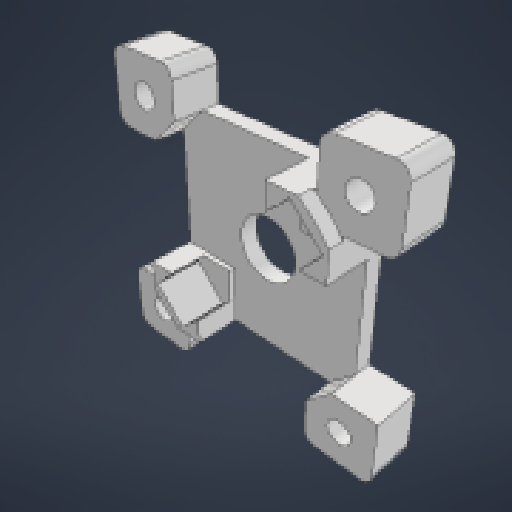
# Autodesk Inventor part: SistemaLiberacion2.2
Saved by Autodesk Inventor 2026.1 (Build 301233000, 233)
## iProperties
Created: 2025-11-13
Part Number: SistemaLiberacion2.2
Material: PLA
Document SubType Name: Modeling
Designer: usuario
Density: 1.3 g/cm^3
Appearance: Genérico
Mass: 76.0734 g
Surface Area: 228.636 cm^2
Volume: 58.518 cm^3
Author: usuario
Autodesk Inventor part; units mm, degrees
ref_plane "YZ Plane" through (0, 0, 0) normal (1, 0, 0) x (0, 1, 0)
ref_plane "XZ Plane" through (0, 0, 0) normal (0, 1, 0) x (-1, 0, 0)
ref_plane "XY Plane" through (0, 0, 0) normal (0, 0, 1) x (1, 0, 0)
sketch "Boceto1" plane through (0, 0, 0) normal (0, 0, 1) x (1, 0, 0)
  line L0 (-49, 49) -> (-49, -49)
  line L1 (-49, -49) -> (49, -49)
  line L2 (49, -49) -> (49, 49)
  line L3 (49, 49) -> (-49, 49)
  line L4 (-49, 49) -> (49, -49) construction
  line L5 (-49, -49) -> (49, 49) construction
  line L6 (-43, 43) -> (-43, -43)
  line L7 (-43, -43) -> (43, -43)
  line L8 (43, -43) -> (43, 43)
  line L9 (43, 43) -> (-43, 43)
  line L10 (-43, 43) -> (43, -43) construction
  line L11 (-43, -43) -> (43, 43) construction
  line L12 (-49, -30) -> (49, -30)
  line L13 (-49, 30) -> (49, 30)
  line L14 (-30, -49) -> (-30, 49)
  line L15 (30, -49) -> (30, 49)
  point P0 (0, 0)
  point P1 (0, -30)
  point P2 (0, -49)
  point P3 (-30, 43)
  point P4 (-43, 30)
  point P5 (30, 43)
  point P6 (43, 30)
  point P7 (30, -43)
  point P8 (43, -30)
  point P9 (-30, -43)
  point P10 (-43, -30)
  dimension "d0" = 98
  dimension "d1" = 98
  dimension "d2" = 6
  dimension "d3" = 6
  dimension "d8" = 19
  dimension "d10" = 19
  dimension "d11" = 19
  dimension "d18" = 19
  constraints: 32 end point, 8 point on line, 6 midpoint, 6 perpendicular, 4 parallel, 1 vertical
  measures "d0" distance of L0.start L0.end
  measures "d1" distance of L1.end L0.end
  measures "d2" distance between parallel lines of L1 L7
  measures "d3" distance between parallel lines of L8 L2
  measures "d8" distance of point (0, -30) point (0, -49)
  measures "d10" distance between parallel lines of L14 L0
  measures "d11" distance between parallel lines of L2 L15
  measures "d18" distance between parallel lines of L3 L13
extrude "Extrusión1" add sketch "Boceto1" against normal blind 34 contours L3 L14 L9 L6 L13 L0 | L12 L6 L7 L14 L1 L0 | L3 L2 L13 L8 L9 L15 | L15 L7 L8 L12 L2 L1
sketch "Boceto2" plane through (0, 0, -34) normal (0, 0, -1) x (-1, 0, 0)
  circle A0 centre (0, 0) radius 10.5
  line L0 (30, -49) -> (49, -49) projected
  line L1 (-49, 49) -> (-49, 30) projected
  line L2 (49, -49) -> (-49, -49)
  line L3 (-49, -49) -> (-49, 49)
  line L4 (-49, 49) -> (49, 49)
  line L5 (49, 49) -> (49, -49)
  line L6 (25, -49) -> (-25, -49)
  line L7 (-25, -49) -> (-25, -33.5)
  line L8 (-25, -33.5) -> (25, -33.5)
  line L9 (25, -33.5) -> (25, -49)
  line L10 (25, -49) -> (-25, -33.5) construction
  line L11 (-25, -49) -> (25, -33.5) construction
  line L12 (49, 0) -> (-49, 0) construction
  line L13 (0, -49) -> (0, 49) construction
  line L14 (33.5, -25) -> (33.5, 25)
  line L15 (49, 25) -> (33.5, -25) construction
  line L16 (49, -25) -> (33.5, -25)
  line L17 (49, 25) -> (49, -25)
  line L18 (49, -25) -> (33.5, 25) construction
  line L19 (33.5, 25) -> (49, 25)
  line L20 (25, 33.5) -> (-25, 33.5)
  line L21 (-25, 49) -> (25, 33.5) construction
  line L22 (25, 49) -> (25, 33.5)
  line L23 (-25, 49) -> (25, 49)
  line L24 (25, 49) -> (-25, 33.5) construction
  line L25 (-25, 33.5) -> (-25, 49)
  line L26 (-33.5, 25) -> (-33.5, -25)
  line L27 (-49, -25) -> (-33.5, 25) construction
  line L28 (-49, 25) -> (-33.5, 25)
  line L29 (-49, -25) -> (-49, 25)
  line L30 (-49, 25) -> (-33.5, -25) construction
  line L31 (-33.5, -25) -> (-49, -25)
  point P0 (0, -41.25)
  point P1 (-25, -49)
  point P2 (49, 0)
  point P3 (41.25, 0)
  point P4 (0, 49)
  point P5 (0, 41.25)
  point P6 (-49, 0)
  point P7 (-41.25, 0)
  dimension "d28" = 21
  dimension "d65" = 50
  dimension "d66" = 15.5
  dimension "d82" = 360
  constraints: 60 end point, 5 midpoint, 4 parallel, 2 horizontal, 2 perpendicular, 1 centre point, 1 coincident, 1 collinear, 1 point on line, 49 other
  measures "d28" diameter of A0
  measures "d65" distance of L7.end L8.end
  measures "d66" distance of L6.end L7.end
extrude "Extrusión2" add sketch "Boceto2" along normal blind 6 contours L2 L9 L8 L7 L3 L31 L26 L28 L1 L4 L25 L20 L22 L5 L19 L14 L16 L0
sketch "Boceto3" plane through (0, 0, -34) normal (0, 0, 1) x (1, 0, 0)
  line L0 (30, -49) -> (-30, -49) projected
  line L1 (-49, -30) -> (-49, 30) projected
  line L2 (-25, -49) -> (-49, -49)
  line L3 (-49, -49) -> (-49, -25)
  line L4 (-49, -25) -> (-33.5, -25)
  line L5 (-25, -33.5) -> (-25, -49)
  line L6 (30, 43) -> (30, 49) projected
  line L7 (25, 49) -> (30, 49) projected
  line L8 (-30, 49) -> (-30, 43) projected
  line L9 (-30, 43) -> (-43, 43) projected
  line L10 (-43, 43) -> (-43, 30) projected
  line L11 (-43, 30) -> (-49, 30) projected
  line L12 (-49, 25) -> (-49, 30) projected
  line L13 (-49, -30) -> (-43, -30) projected
  line L14 (-43, -30) -> (-43, -43) projected
  line L15 (-43, -43) -> (-30, -43) projected
  line L16 (-30, -43) -> (-30, -49) projected
  line L17 (-25, -49) -> (-30, -49) projected
  line L18 (30, -49) -> (30, -43) projected
  line L19 (30, -43) -> (43, -43) projected
  line L20 (43, -43) -> (43, -30) projected
  line L21 (43, -30) -> (49, -30) projected
  line L22 (49, -25) -> (49, -30) projected
  line L23 (49, 30) -> (43, 30) projected
  line L24 (43, 30) -> (43, 43) projected
  line L25 (43, 43) -> (30, 43) projected
  circle A0 centre (0, 0) radius 10.5 projected
  line L26 (-25, -33.5) -> (-13.5, -33.5)
  line L27 (-13.5, -33.5) -> (-13.5, -13.5)
  line L28 (-13.5, -13.5) -> (-33.5, -13.5)
  line L29 (-33.5, -13.5) -> (-33.5, -25)
  line L30 (-13.5, -29.5) -> (-29.5, -13.5)
  circle A1 centre (0, 0) radius 10.5 projected
  line L31 (13.5, 13.5) -> (33.5, 13.5)
  line L32 (13.5, 33.5) -> (13.5, 13.5)
  line L33 (13.5, 29.5) -> (29.5, 13.5)
  line L34 (33.5, 13.5) -> (33.5, 25)
  line L35 (25, 33.5) -> (13.5, 33.5)
  line L36 (25, 49) -> (49, 49)
  line L37 (49, 49) -> (49, 25)
  line L38 (49, 25) -> (33.5, 25)
  line L39 (25, 33.5) -> (25, 49)
  line L40 (25, 33.5) -> (25, 49) projected
  line L41 (-25, 33.5) -> (25, 33.5) projected
  line L42 (-25, 49) -> (-25, 33.5) projected
  line L43 (-30, 49) -> (-25, 49) projected
  line L44 (-33.5, 25) -> (-49, 25) projected
  line L45 (-33.5, -25) -> (-33.5, 25) projected
  line L46 (-49, -25) -> (-33.5, -25) projected
  line L47 (-49, -30) -> (-49, -25) projected
  line L48 (-25, -33.5) -> (-25, -49) projected
  line L49 (25, -33.5) -> (-25, -33.5) projected
  line L50 (25, -49) -> (25, -33.5) projected
  line L51 (30, -49) -> (25, -49) projected
  line L52 (33.5, -25) -> (49, -25) projected
  line L53 (33.5, 25) -> (33.5, -25) projected
  line L54 (49, 25) -> (33.5, 25) projected
  line L55 (49, 30) -> (49, 25) projected
  line L56 (-49, -30) -> (-49, -49) projected
  line L57 (33.5, -25) -> (25, -33.5)
  line L58 (-25, 33.5) -> (-33.5, 25)
  point P0 (49, 49)
  point P1 (30, 49)
  point P2 (49, 30)
  point P3 (49, 25)
  point P4 (49, 30)
  point P5 (43, 30)
  point P6 (43, 43)
  point P7 (30, 43)
  point P8 (30, 49)
  dimension "d74" = 4
  dimension "d77" = 360
  dimension "d84" = 45
  dimension "d85" = 20
  dimension "d86" = 20
  constraints: 40 end point, 4 collinear, 4 parallel, 4 point on line, 2 horizontal, 2 perpendicular, 53 other
  measures "d74" distance of L28.end L30.end
  measures "d84" angle of L30 L45
  measures "d85" distance of L26.end L27.end
  measures "d86" distance of L27.end L28.end
extrude "Extrusión3" add sketch "Boceto3" along normal blind 15 contours L0 L50 L57 L52 L22 L21 L20 L19 L18 | L0 L16 L15 L14 L13 L1 L4 L29 L28 L30 L27 L26 L5 | L30 L28 L27 | L31 L33 L32 L35 L39 L7 L6 L25 L24 L23 L37 L38 L34 | L31 L32 L33 | L1 L11 L10 L9 L8 L43 L42 L58 L44
sketch "Boceto4" plane through (0, 0, -19) normal (0, 0, 1) x (1, 0, 0)
  line L0 (30, 49) -> (30, 43) projected
  line L1 (43, 43) -> (43, 30) projected
  line L2 (30, 43) -> (43, 43) projected
  line L3 (-18.7383, -7.4246) -> (-27.9307, -16.617)
  line L4 (-27.9307, -16.617) -> (-16.617, -27.9307)
  line L5 (-16.617, -27.9307) -> (-7.4246, -18.7383)
  line L6 (-7.4246, -18.7383) -> (-18.7383, -7.4246)
  line L7 (-16.617, -27.9307) -> (-18.7383, -7.4246) construction
  line L8 (-27.9307, -16.617) -> (-7.4246, -18.7383) construction
  circle A0 centre (0, 0) radius 10.5 construction
  line L9 (18.7383, 7.4246) -> (27.9307, 16.617)
  line L10 (27.9307, 16.617) -> (16.617, 27.9307)
  line L11 (16.617, 27.9307) -> (18.7383, 7.4246) construction
  line L12 (27.9307, 16.617) -> (7.4246, 18.7383) construction
  line L13 (7.4246, 18.7383) -> (18.7383, 7.4246)
  line L14 (16.617, 27.9307) -> (7.4246, 18.7383)
  line L15 (49, -49) -> (25, -49) construction
  line L16 (-49, -49) -> (-49, 49) construction
  line L17 (49, -49) -> (-49, -49) construction
  line L18 (-49, -49) -> (-49, 49) construction
  line L19 (-49, 49) -> (49, 49) construction
  line L20 (49, 49) -> (49, -49) construction
  line L21 (49, -49) -> (-49, -49) construction
  line L22 (49, 49) -> (-49, -49) construction
  line L23 (-49, 49) -> (49, -49) construction
  point P0 (0, 0)
  point P1 (-17.6777, -17.6777)
  point P2 (17.6777, 17.6777)
  point P3 (-17.6777, -17.6777)
  point P4 (-49, 25)
  point P5 (-25, -49)
  dimension "d54" = 13
  dimension "d57" = 16
  dimension "d61" = 360
  dimension "d64" = 25
  dimension "d79" = 8
  constraints: 36 end point, 4 perpendicular, 2 midpoint, 2 parallel, 1 coincident, 1 horizontal, 1 point on line, 23 other
  measures "d54" distance of L3.start L3.end
  measures "d57" distance of L3.end L4.end
  measures "d64" distance of point (0, 0) point (-17.678, -17.678)
  measures "d79" distance between parallel lines of L22 L3
extrude "Extrusión4" cut sketch "Boceto4" against normal blind 13
sketch "Boceto6" plane through (0, 0, 0) normal (0, 0, 1) x (1, 0, 0)
  line L0 (-49, -49) -> (-30, -49) projected
  line L1 (-49, -30) -> (-49, -49) projected
  line L2 (-49, 49) -> (-49, 30) projected
  line L3 (-30, 49) -> (-49, 49) projected
  line L4 (49, 49) -> (30, 49) projected
  line L5 (49, 30) -> (49, 49) projected
  line L6 (30, -49) -> (49, -49) projected
  line L7 (49, -49) -> (49, -30) projected
  line L8 (-43, -43) -> (-43, -30) projected
  line L9 (-30, -43) -> (-43, -43) projected
  line L10 (-43, 30) -> (-43, 43) projected
  line L11 (-43, 43) -> (-30, 43) projected
  line L12 (30, 43) -> (43, 43) projected
  line L13 (43, 43) -> (43, 30) projected
  line L14 (43, -30) -> (43, -43) projected
  line L15 (43, -43) -> (30, -43) projected
  line L16 (-43, -43) -> (43, -43)
  line L17 (43, -43) -> (43, 43)
  line L18 (43, 43) -> (-43, 43)
  line L19 (-43, 43) -> (-43, -43)
  line L20 (-49, -49) -> (49, -49)
  line L21 (49, -49) -> (49, 49)
  line L22 (49, 49) -> (-49, 49)
  line L23 (-49, 49) -> (-49, -49)
  point P0 (0, 0)
  constraints: 16 end point, 4 parallel, 2 horizontal, 2 perpendicular
extrude "Extrusión5" cut sketch "Boceto6" against normal blind 11
sketch "Boceto8" plane through (0, 0, -19) normal (0, 0, 1) x (1, 0, 0)
  line L0 (-49, 49) -> (-25, 49) construction
  line L1 (49, -49) -> (25, -49) construction
  line L2 (-49, 49) -> (49, 49) construction
  line L3 (49, 49) -> (49, -49) construction
  line L4 (49, -49) -> (-49, -49) construction
  line L5 (-49, -49) -> (-49, 49) construction
  line L6 (-49, 49) -> (49, -49) construction
  line L7 (49, 49) -> (-49, -49) construction
  line L8 (-27.6832, -16.8645) -> (-31.9259, -21.1071)
  line L9 (-31.9259, -21.1071) -> (-21.1071, -31.9259)
  line L10 (-27.6832, -16.8645) -> (-16.8645, -27.6832)
  line L11 (-16.8645, -27.6832) -> (-21.1071, -31.9259)
  line L12 (-27.6832, -16.8645) -> (-21.1071, -31.9259) construction
  line L13 (-31.9259, -21.1071) -> (-16.8645, -27.6832) construction
  line L14 (-16.617, -27.9307) -> (-27.9307, -16.617) construction
  line L15 (-31.9259, -21.1071) -> (-23.4406, -12.6219) construction
  line L16 (-23.4406, -12.6219) -> (-12.6219, -23.4406) construction
  line L17 (-12.6219, -23.4406) -> (-21.1071, -31.9259) construction
  circle A0 centre (0, 0) radius 10.5 projected
  line L18 (27.6832, 16.8645) -> (16.8645, 27.6832)
  line L19 (31.9259, 21.1071) -> (16.8645, 27.6832) construction
  line L20 (31.9259, 21.1071) -> (21.1071, 31.9259)
  line L21 (27.6832, 16.8645) -> (21.1071, 31.9259) construction
  line L22 (16.8645, 27.6832) -> (21.1071, 31.9259)
  line L23 (27.6832, 16.8645) -> (31.9259, 21.1071)
  point P0 (-24.3952, -24.3952)
  point P1 (24.3952, 24.3952)
  point P2 (23.4406, 12.6219)
  dimension "d87" = 6
  dimension "d88" = 15.3
  dimension "d89" = 12
  dimension "d94" = 360
  constraints: 42 end point, 4 parallel, 4 perpendicular, 3 point on line, 2 collinear, 1 horizontal, 1 midpoint, 25 other
  measures "d87" distance of L8.start L8.end
  measures "d88" distance of L8.end L9.end
  measures "d89" distance of L8.end L15.end
extrude "Extrusión7" cut sketch "Boceto8" against normal blind 18 contours L10 L11 L9 L8 | L18 L22 L20 L23
sketch "Boceto9" plane through (0, 0, -19) normal (0, 0, 1) x (1, 0, 0)
  circle A0 centre (37, -37) radius 4.15
  circle A1 centre (0, 0) radius 10.5 projected
  line L0 (49, -25) -> (49, -49) projected
  line L1 (49, -49) -> (25, -49)
  line L2 (49, -25) -> (49, -49)
  line L3 (49, -25) -> (33.5, -25) projected
  line L4 (49, -49) -> (25, -49)
  line L5 (25, -49) -> (25, -25)
  line L6 (25, -25) -> (49, -25)
  line L7 (49, -25) -> (49, -49)
  line L8 (25, -33.5) -> (25, -49) projected
  line L9 (25, -49) -> (49, -25) construction
  line L10 (49, -49) -> (25, -25) construction
  circle A2 centre (37, 37) radius 4.15
  line L11 (49, 49) -> (49, 25)
  line L12 (25, 49) -> (49, 49)
  line L13 (49, 49) -> (49, 25)
  line L14 (49, 25) -> (25, 25)
  line L15 (25, 25) -> (25, 49)
  line L16 (25, 49) -> (49, 49)
  line L17 (49, 25) -> (25, 49) construction
  line L18 (49, 49) -> (25, 25) construction
  circle A3 centre (-37, 37) radius 4.15
  line L19 (-49, 49) -> (-25, 49)
  line L20 (-49, 25) -> (-49, 49)
  line L21 (-49, 49) -> (-25, 49)
  line L22 (-25, 49) -> (-25, 25)
  line L23 (-25, 25) -> (-49, 25)
  line L24 (-49, 25) -> (-49, 49)
  line L25 (-25, 49) -> (-49, 25) construction
  line L26 (-49, 49) -> (-25, 25) construction
  circle A4 centre (-37, -37) radius 4.15
  line L27 (-49, -49) -> (-49, -25)
  line L28 (-25, -49) -> (-49, -49)
  line L29 (-49, -49) -> (-49, -25)
  line L30 (-49, -25) -> (-25, -25)
  line L31 (-25, -25) -> (-25, -49)
  line L32 (-25, -49) -> (-49, -49)
  line L33 (-49, -25) -> (-25, -49) construction
  line L34 (-49, -49) -> (-25, -25) construction
  point P0 (25, 49)
  point P1 (33.5, 25)
  point P2 (25, 33.5)
  point P3 (-49, 25)
  point P4 (-25, 33.5)
  point P5 (-33.5, 25)
  point P6 (-25, -49)
  point P7 (-33.5, -25)
  point P8 (-25, -33.5)
  dimension "d98" = 8.3
  dimension "d115" = 360
  constraints: 64 end point, 4 centre point, 2 collinear, 2 horizontal, 2 parallel, 2 perpendicular, 1 midpoint, 77 other
  measures "d98" diameter of A0
extrude "Extrusión8" cut sketch "Boceto9" against normal up to next contours A0 | A2 | A3 | A4
sketch "Boceto11" plane through (0, 0, -11) normal (0, 0, 1) x (1, 0, 0)
  circle A0 centre (0, 0) radius 41
  circle A1 centre (0, 0) radius 10.5 projected
  line L0 (-49, 30) -> (-49, 25) projected
  line L1 (-49, 25) -> (-33.5, 25) projected
  line L2 (-33.5, 25) -> (-25, 33.5) projected
  line L3 (-25, 33.5) -> (-25, 49) projected
  line L4 (-25, 49) -> (-30, 49) projected
  line L5 (-30, 43) -> (-30, 49) projected
  line L6 (-43, 43) -> (-30, 43) projected
  line L7 (-43, 30) -> (-43, 43) projected
  line L8 (-49, 30) -> (-43, 30) projected
  line L9 (-30, 49) -> (-30, 43) projected
  line L10 (-49, 49) -> (-30, 49) projected
  line L11 (-49, 30) -> (-49, 49) projected
  line L12 (-43, 30) -> (-49, 30) projected
  line L13 (-43, 43) -> (-43, 30) projected
  line L14 (-30, 43) -> (-43, 43) projected
  line L15 (49, 30) -> (43, 30) projected
  line L16 (49, 49) -> (49, 30) projected
  line L17 (30, 49) -> (49, 49) projected
  line L18 (30, 43) -> (30, 49) projected
  line L19 (43, 43) -> (30, 43) projected
  line L20 (43, 30) -> (43, 43) projected
  line L21 (16.8645, 27.6832) -> (21.1071, 31.9259) projected
  line L22 (21.1071, 31.9259) -> (31.9259, 21.1071) projected
  line L23 (31.9259, 21.1071) -> (27.6832, 16.8645) projected
  line L24 (27.6832, 16.8645) -> (27.9307, 16.617) projected
  line L25 (27.9307, 16.617) -> (24.8137, 13.5) projected
  line L26 (24.8137, 13.5) -> (33.5, 13.5) projected
  line L27 (33.5, 13.5) -> (33.5, 25) projected
  line L28 (33.5, 25) -> (49, 25) projected
  line L29 (49, 25) -> (49, 30) projected
  line L30 (43, 30) -> (49, 30) projected
  line L31 (43, 43) -> (43, 30) projected
  line L32 (30, 43) -> (43, 43) projected
  line L33 (30, 49) -> (30, 43) projected
  line L34 (30, 49) -> (25, 49) projected
  line L35 (25, 49) -> (25, 33.5) projected
  line L36 (25, 33.5) -> (13.5, 33.5) projected
  line L37 (13.5, 33.5) -> (13.5, 24.8137) projected
  line L38 (13.5, 24.8137) -> (16.617, 27.9307) projected
  line L39 (16.617, 27.9307) -> (16.8645, 27.6832) projected
  circle A2 centre (37, -37) radius 4.15 projected
  line L40 (43, -43) -> (30, -43) projected
  line L41 (43, -30) -> (43, -43) projected
  line L42 (49, -30) -> (43, -30) projected
  line L43 (49, -30) -> (49, -25) projected
  line L44 (49, -25) -> (33.5, -25) projected
  line L45 (33.5, -25) -> (25, -33.5) projected
  line L46 (25, -33.5) -> (25, -49) projected
  line L47 (25, -49) -> (30, -49) projected
  line L48 (30, -43) -> (30, -49) projected
  line L49 (30, -49) -> (30, -43) projected
  line L50 (49, -49) -> (30, -49) projected
  line L51 (49, -30) -> (49, -49) projected
  line L52 (43, -30) -> (49, -30) projected
  line L53 (43, -43) -> (43, -30) projected
  line L54 (30, -43) -> (43, -43) projected
  line L55 (-30, -43) -> (-30, -49) projected
  line L56 (-43, -43) -> (-30, -43) projected
  line L57 (-43, -30) -> (-43, -43) projected
  line L58 (-49, -30) -> (-43, -30) projected
  line L59 (-49, -49) -> (-49, -30) projected
  line L60 (-30, -49) -> (-49, -49) projected
  line L61 (-31.9259, -21.1071) -> (-27.6832, -16.8645) projected
  line L62 (-27.6832, -16.8645) -> (-27.9307, -16.617) projected
  line L63 (-27.9307, -16.617) -> (-24.8137, -13.5) projected
  line L64 (-24.8137, -13.5) -> (-33.5, -13.5) projected
  line L65 (-33.5, -13.5) -> (-33.5, -25) projected
  line L66 (-33.5, -25) -> (-49, -25) projected
  line L67 (-49, -25) -> (-49, -30) projected
  line L68 (-43, -30) -> (-49, -30) projected
  line L69 (-43, -43) -> (-43, -30) projected
  line L70 (-30, -43) -> (-43, -43) projected
  line L71 (-30, -49) -> (-30, -43) projected
  line L72 (-30, -49) -> (-25, -49) projected
  line L73 (-25, -49) -> (-25, -33.5) projected
  line L74 (-25, -33.5) -> (-13.5, -33.5) projected
  line L75 (-13.5, -33.5) -> (-13.5, -24.8137) projected
  line L76 (-13.5, -24.8137) -> (-16.617, -27.9307) projected
  line L77 (-16.617, -27.9307) -> (-16.8645, -27.6832) projected
  line L78 (-16.8645, -27.6832) -> (-21.1071, -31.9259) projected
  line L79 (-21.1071, -31.9259) -> (-31.9259, -21.1071) projected
  line L80 (-33.5, -13.5) -> (-33.5, 25) projected
  line L81 (33.5, 25) -> (33.5, -25) projected
  line L82 (-25, 33.5) -> (13.5, 33.5) projected
  line L83 (25, -33.5) -> (-25, -33.5) projected
  line L84 (-49, 49) -> (49, 49)
  line L85 (49, 49) -> (49, -49)
  line L86 (49, -49) -> (-49, -49)
  line L87 (-49, -49) -> (-49, 49)
  dimension "d112" = 82
  constraints: 8 end point, 2 collinear, 2 parallel, 1 centre point, 1 coincident, 1 horizontal, 1 perpendicular
  measures "d112" diameter of A0
extrude "Extrusión9" cut sketch "Boceto11" against normal blind 13 contours A0 L27 L28 L85 L44 L81 | A0 L36 L35 L34 L18 L19 L20 L15 L29 L28 L27 | L81 L45 L83 A0 | A0 L82 L3 L84 L35 L36 | L83 L46 L86 L73 L74 A0 | L44 L43 L42 L41 L40 L48 L47 L46 L45 | A0 L80 L2 L82 | L74 L73 L72 L55 L56 L57 L58 L67 L66 L65 A0 | A0 L65 L66 L87 L1 L80 | L2 L1 L0 L8 L7 L6 L5 L4 L3 | L15 L20 L19 L18 L17 L16 | L51 L50 L48 L40 L41 L42 | L5 L6 L7 L8 L11 L10 | L60 L59 L58 L57 L56 L55
fillet "Empalme1" radius 4 11 edges at (-49, -49, -32) (49, -49, -32) (49, 49, -32) (-49, 49, -32) (-25, -49, -32) (25, -49, -32) (-49, -25, -32) (-49, 25, -32) (-25, 49, -32) (25, 49, -32) (49, 25, -32)
